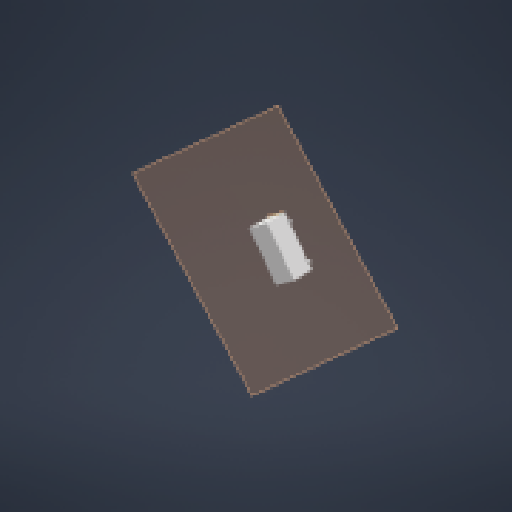
# Autodesk Inventor part: Battery_Holder
Saved by Autodesk Inventor 2024.2 (Build 282272000, 272)
## iProperties
Created: 2024-03-31
Part Number: Battery_Holder
Material: Generic
Document SubType Name: Modeling
Designer: warm
Density: 1 g/cm^3
Appearance: Default
Author: warm
Autodesk Inventor part; units mm, degrees
ref_plane "YZ Plane" through (0, 0, 0) normal (1, 0, 0) x (0, 1, 0)
ref_plane "XZ Plane" through (0, 0, 0) normal (0, 1, 0) x (-1, 0, 0)
ref_plane "XY Plane" through (0, 0, 0) normal (0, 0, 1) x (1, 0, 0)
ref_plane "Work Plane1" through (-774.147, 14.6804, 0) normal (0, 0, -1) x (0.5974542, -0.801903, 0)
sketch "Sketch1" plane through (-774.147, 14.6804, 0) normal (0, 0, -1) x (0.5974542, -0.801903, 0)
  line L0 (58.7225, -26.2361) -> (-57.2775, -26.2361)
  line L1 (-57.2775, -26.2361) -> (-57.2775, 25.7639)
  line L2 (-57.2775, 25.7639) -> (58.7225, 25.7639)
  line L3 (58.7225, 25.7639) -> (58.7225, -26.2361)
  arc A0 (19.6988, -21.7639) -> (2.3103, -21.7639) centre (11.0046, -62.2541) ccw construction
  arc A1 (19.6988, -21.7639) -> (24.3194, -21.7639) centre (22.0091, -11.0045) ccw construction
  arc A2 (41.7079, -21.7639) -> (24.3194, -21.7639) centre (33.0137, -62.2541) ccw construction
  arc A3 (41.7079, -21.7639) -> (54.7775, -8.6943) centre (44.0182, -11.0045) ccw construction
  arc A4 (54.7775, 8.6943) -> (54.7775, -8.6943) centre (95.2678, 0) ccw construction
  arc A5 (54.7775, 8.6943) -> (41.7079, 21.7639) centre (44.0182, 11.0046) ccw construction
  arc A6 (24.3194, 21.7639) -> (41.7079, 21.7639) centre (33.0137, 62.2541) ccw construction
  arc A7 (24.3194, 21.7639) -> (19.6988, 21.7639) centre (22.0091, 11.0046) ccw construction
  arc A8 (2.3103, 21.7639) -> (19.6988, 21.7639) centre (11.0046, 62.2541) ccw construction
  arc A9 (2.3103, 21.7639) -> (-2.3103, 21.7639) centre (0, 11.0046) ccw construction
  arc A10 (-19.6988, 21.7639) -> (-2.3103, 21.7639) centre (-11.0045, 62.2541) ccw construction
  arc A11 (-19.6988, 21.7639) -> (-24.3194, 21.7639) centre (-22.0091, 11.0046) ccw construction
  arc A12 (-41.7079, 21.7639) -> (-24.3194, 21.7639) centre (-33.0136, 62.2541) ccw construction
  arc A13 (-41.7079, 21.7639) -> (-54.7775, 8.6943) centre (-44.0182, 11.0046) ccw construction
  arc A14 (-54.7775, -8.6943) -> (-54.7775, 8.6943) centre (-95.2678, 0) ccw construction
  arc A15 (-54.7775, -8.6943) -> (-41.7079, -21.7639) centre (-44.0182, -11.0045) ccw construction
  arc A16 (-24.3194, -21.7639) -> (-41.7079, -21.7639) centre (-33.0136, -62.2541) ccw construction
  arc A17 (-24.3194, -21.7639) -> (-19.6988, -21.7639) centre (-22.0091, -11.0045) ccw construction
  arc A18 (-2.3103, -21.7639) -> (-19.6988, -21.7639) centre (-11.0045, -62.2541) ccw construction
  arc A19 (-2.3103, -21.7639) -> (2.3103, -21.7639) centre (0, -11.0045) ccw construction
  line L4 (159.874, 0.748) -> (161.144, 0.748) construction
  line L5 (161.144, 0.748) -> (161.144, -3.697) construction
  line L6 (159.874, -3.697) -> (161.144, -3.697) construction
  line L7 (159.874, -3.697) -> (159.874, 0.748) construction
  line L8 (63.7225, -31.2361) -> (-62.2775, -31.2361)
  line L9 (-62.2775, -31.2361) -> (-62.2775, 30.7639)
  line L10 (-62.2775, 30.7639) -> (63.7225, 30.7639)
  line L11 (63.7225, 30.7639) -> (63.7225, -31.2361)
  line L12 (58.7225, -26.2361) -> (63.7225, -26.2361)
  line L13 (-57.2775, -26.2361) -> (-62.2775, -26.2361)
  line L14 (-57.2775, 25.7639) -> (-62.2775, 25.7639)
  line L15 (58.7225, 25.7639) -> (63.7225, 25.7639)
  point P0 (474.2897, -612.02)
  dimension "d0" = 116
  dimension "d1" = 52
  dimension "d2" = 2.5
  dimension "d3" = 4
  dimension "d4" = 5
  constraints: 40 point on circle, 32 end point, 20 centre point, 6 point on line, 4 parallel, 4 perpendicular, 3 horizontal, 2 vertical, 67 other
  measures "d0" distance of L1.end L2.end
  measures "d1" distance of L0.end L1.end
  measures "d2" distance from line of A14.start L1
  measures "d3" distance from line of A11.end L2
  measures "d4" distance between parallel lines of L3 L11
extrude "Extrusion1" add sketch "Sketch1" against normal blind 47 contours L12 L11 L8 L9 L13 L0 | L13 L9 L14 L1 | L2 L14 L9 L10 L11 L15
sketch "Sketch2" plane through (-774.147, 14.6804, 47) normal (0, 0, 1) x (0.5974542, -0.801903, 0)
  line L0 (-62.2775, -30.7639) -> (63.7225, -30.7639) projected
  line L1 (63.7225, 31.2361) -> (-62.2775, 31.2361) projected
  line L2 (63.7225, -30.7639) -> (-62.2775, -30.7639)
  line L3 (-62.2775, -30.7639) -> (-62.2775, 31.2361)
  line L4 (-62.2775, 31.2361) -> (63.7225, 31.2361)
  line L5 (63.7225, 31.2361) -> (63.7225, -30.7639)
  point P0 (474.2897, 612.02)
  point P1 (-62.2775, -30.7639)
  point P2 (63.7225, 31.2361)
  constraints: 8 end point, 2 parallel, 1 horizontal, 1 perpendicular
extrude "Extrusion2" add sketch "Sketch2" along normal blind 3
fillet "Fillet1" radius 1.5875 6 edges at (-711.0274, -17.7567, 25) (-786.3067, 83.283, 25) (-760.7454, -54.7989, 25) (-756.7359, -51.8116, 23.5) (-715.037, -20.744, 23.5) (-836.0247, 46.2409, 25)
ref_plane "Work Plane2" through (-841.5049, -36.3773, 0) normal (0, 0, 1) x (0.6694225, -0.7428819, 0)
sketch "Sketch3" plane through (-841.5049, -36.3773, 0) normal (0, 0, 1) x (0.6694225, -0.7428819, 0)
  line L0 (-50.362, 120.9615) -> (71.931, 109.5419) projected
  line L1 (66.1667, 47.8105) -> (-56.1263, 59.23) projected
  line L2 (73.3641, 107.8137) -> (73.1944, 105.9966) projected
  line L3 (-57.5594, 60.9582) -> (-52.0902, 119.5284) projected
  circle A0 centre (-39.2118, 52.5485) radius 2.15
  circle A1 centre (48.3075, 44.3761) radius 2.15
  line L4 (68.0646, 51.0606) -> (67.8949, 49.2435) projected
  arc A2 (-44.0243, 54.1752) -> (-34.1813, 53.2561) centre (-39.2118, 52.5485) ccw
  line L5 (40.7824, 50.1808) -> (48.7798, 49.434)
  arc A3 (-44.0243, 54.1752) -> (-46.7369, 58.3532) centre (-47.0321, 55.192) ccw
  arc A4 (-30.7421, 56.8597) -> (-34.1813, 53.2561) centre (-31.0373, 53.6984) ccw
  arc A5 (43.495, 46.0028) -> (53.338, 45.0837) centre (48.3075, 44.3761) ccw
  arc A6 (43.495, 46.0028) -> (40.7824, 50.1808) centre (40.4872, 47.0196) ccw
  arc A7 (43.495, 46.0028) -> (40.7824, 50.1808) centre (40.4872, 47.0196) ccw
  line L6 (66.1667, 47.8105) -> (40.7824, 50.1808)
  arc A8 (43.495, 46.0028) -> (40.7824, 50.1808) centre (40.4872, 47.0196) ccw
  line L7 (48.3075, 44.3761) -> (48.6282, 47.8105)
  arc A9 (56.7772, 48.6873) -> (53.338, 45.0837) centre (56.482, 45.526) ccw
  line L8 (-54.8248, 90.2433) -> (-8.2036, 85.8899) construction
  line L9 (71.931, 109.5419) -> (-50.362, 120.9615)
  circle A10 centre (-32.5028, 124.3959) radius 2.15
  circle A11 centre (55.0165, 116.2235) radius 2.15
  line L10 (73.1944, 105.9966) -> (73.3641, 107.8137)
  arc A12 (-27.6903, 122.7691) -> (-37.5332, 123.6882) centre (-32.5028, 124.3959) ccw
  line L11 (46.5468, 111.9123) -> (54.5442, 111.1655)
  arc A13 (-40.9725, 120.0847) -> (-37.5332, 123.6882) centre (-40.6773, 123.2459) ccw
  arc A14 (-27.6903, 122.7691) -> (-24.9777, 118.5911) centre (-24.6825, 121.7524) ccw
  arc A15 (59.829, 114.5967) -> (49.986, 115.5158) centre (55.0165, 116.2235) ccw
  arc A16 (46.5468, 111.9123) -> (49.986, 115.5158) centre (46.842, 115.0735) ccw
  arc A17 (46.5468, 111.9123) -> (49.986, 115.5158) centre (46.842, 115.0735) ccw
  line L12 (71.931, 109.5419) -> (46.5468, 111.9123)
  arc A18 (46.5468, 111.9123) -> (49.986, 115.5158) centre (46.842, 115.0735) ccw
  line L13 (55.0165, 116.2235) -> (54.6958, 112.7891)
  arc A19 (59.829, 114.5967) -> (62.5416, 110.4187) centre (62.8368, 113.58) ccw
  point P0 (536.2982, 649.4905)
  point P1 (73.2792, 106.9052)
  point P2 (48.7798, 49.434)
  point P3 (54.5442, 111.1655)
  point P4 (-40.9725, 120.0847)
  point P5 (-24.9777, 118.5911)
  point P6 (49.986, 115.5158)
  point P7 (46.5468, 111.9123)
  point P8 (62.5416, 110.4187)
  point P9 (43.495, 46.0028)
  point P10 (56.7772, 48.6873)
  point P11 (40.7824, 50.1808)
  point P12 (-30.7421, 56.8597)
  point P13 (-46.7369, 58.3532)
  dimension "d16" = 4.3
  dimension "d18" = 4.3
  dimension "d20" = 19.05
  dimension "d21" = 19.05
  dimension "d24" = 5.08
  dimension "d25" = 3.175
  dimension "d26" = 3.175
  dimension "d27" = 3.175
  dimension "d28" = 5.08
  dimension "d29" = 3.175
  dimension "d30" = 3.175
  constraints: 38 point on circle, 28 symmetric about line, 20 centre point, 18 end point, 14 point on line, 12 tangent, 4 coincident, 2 collinear, 2 midpoint, 2 perpendicular, 11 other
  measures "d16" diameter of A0
  measures "d18" diameter of A1
  measures "d20" distance from line of L3 A0.centre
  measures "d21" distance from line of L4 A1.centre
  measures "d24" distance from line of L1 A0.centre
  measures "d25" radius of A3
  measures "d26" radius of A4
  measures "d27" radius of A6
  measures "d28" distance from line of L1 L7.start
  measures "d29" radius of A7
  measures "d30" radius of A8
extrude "Extrusion3" add sketch "Sketch3" along normal blind 3
body "Solid1"
